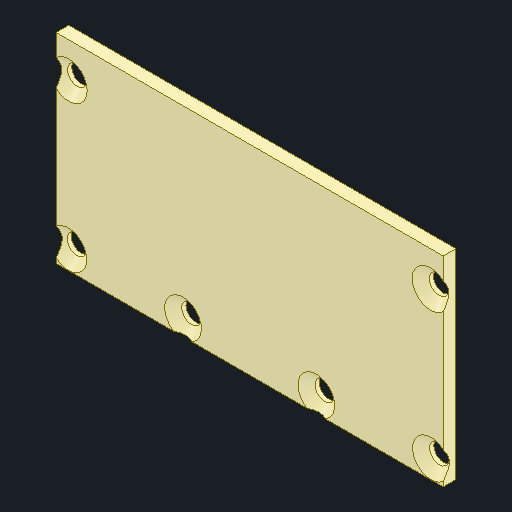
# Autodesk Inventor part: back
Saved by Autodesk Inventor 2023 (Build 270158000, 158)
## iProperties
Created: 2024-05-19
Part Number: back
Material: Nylon 6/6
Document SubType Name: Modeling
Designer: szymo
Density: 1.13 g/cm^3
Appearance: Nylon 6
Mass: 3.55753 g
Surface Area: 44.8899 cm^2
Volume: 3.14826 cm^3
Author: szymo
Autodesk Inventor part; units mm, degrees
ref_plane "YZ Plane" through (0, 0, 0) normal (1, 0, 0) x (0, 1, 0)
ref_plane "XZ Plane" through (0, 0, 0) normal (0, 1, 0) x (-1, 0, 0)
ref_plane "XY Plane" through (0, 0, 0) normal (0, 0, 1) x (1, 0, 0)
ref_plane "Work Plane1" through (22, 31.5, 0) normal (0, 0, 1) x (0, 1, 0)
sketch "Sketch1" plane through (22, 31.5, 0) normal (0, 0, 1) x (0, 1, 0)
  line L0 (0, 0) -> (0, 61) projected
  line L1 (0, 61) -> (-3.5, 61) projected
  line L2 (-3.5, 0) -> (-3.5, 61) projected
  circle A0 centre (-5.5, 2) radius 1.75 projected
  circle A1 centre (-28.5, 2) radius 1.75 projected
  line L3 (-3.5, 4) -> (-7.5, 4) projected
  arc A2 (-8.5, 3) -> (-7.5, 4) centre (-8.5, 4) ccw projected
  line L4 (-8.5, 3) -> (-21.7679, 3) projected
  arc A3 (-23.5, 4) -> (-21.7679, 3) centre (-21.7679, 5) ccw projected
  line L5 (-23.5, 4) -> (-31.5, 4) projected
  line L6 (-31.5, 0) -> (-31.5, 4) projected
  line L7 (-3.5, 0) -> (-3.5, 4) projected
  line L8 (-23.5, 22) -> (-3.5, 22) projected
  line L9 (-3.5, 22) -> (-3.5, 18) projected
  line L10 (-23.5, 39) -> (-3.5, 39) projected
  line L11 (-3.5, 39) -> (-3.5, 43) projected
  line L12 (-3.5, 57) -> (-6.7679, 57) projected
  line L13 (-3.5, 61) -> (-3.5, 57) projected
  line L14 (-3.5, 61) -> (-31.5, 61) projected
  line L15 (-31.5, 61) -> (-31.5, 57) projected
  line L16 (-24.004, 57) -> (-31.5, 57) projected
  line L17 (0, 0) -> (-31.5, 0)
  line L18 (-31.5, 0) -> (-31.5, 61)
  line L19 (-31.5, 61) -> (0, 61)
  line L20 (0, 61) -> (0, 0)
  line L21 (-3.5, 0) -> (-31.5, 0)
  line L22 (-8.5, 58) -> (-21.7679, 58) projected
  arc A4 (-7.634, 57.5) -> (-6.7679, 57) centre (-6.7679, 58) ccw projected
  arc A5 (-24.004, 57) -> (-23.2587, 57.3333) centre (-24.004, 58) ccw projected
  arc A6 (-21.7679, 58) -> (-23.2587, 57.3333) centre (-21.7679, 56) ccw projected
  arc A7 (-7.634, 57.5) -> (-8.5, 58) centre (-8.5, 57) ccw projected
  line L23 (-23.5, 18) -> (-23.5, 22) projected
  line L24 (-23.5, 18) -> (-3.5, 18) projected
  line L25 (-23.5, 43) -> (-3.5, 43) projected
  line L26 (-23.5, 43) -> (-23.5, 39) projected
  circle A8 centre (-5.5, 59) radius 1.75 projected
  circle A9 centre (-28.5, 59) radius 1.75 projected
  point P0 (-3.5, 28.5)
  point P1 (-3.5, 32.5)
  point P2 (-3.5, 61)
  point P3 (-13.5, 58)
  dimension "d25" = 0
  dimension "d26" = 0
  constraints: 10 end point, 1 horizontal, 1 parallel, 1 perpendicular, 1 vertical, 1 other
  measures "d25" distance between parallel lines of L19 L1
  measures "d26" distance from line of point (-3.5, 0) L17
extrude "Extrusion1" add sketch "Sketch1" along normal blind 2 contours L17 L2 L1 L0 | L17 L6 L5 A3 L4 A2 L3 L2 | L2 L12 A4 A7 L22 A6 A5 L16 L15 L14 | L3 A2 L4 A3 L5 L18 L16 A5 A6 L22 A7 A4 L12 L2 L25 L26 L10 L8 L23 L24 | L24 L23 L8 L2 | L2 L10 L26 L25 | A0 | A1 | A8 | A9
hole "Hole1" at (20.0645, 2.9032, 2) at (20, 26, 2) at (2, 2.5, 2) at (-19, 2.5, 2) at (-37, 26, 2) at (-37.0645, 2.9032, 2) direction (0, 0, -1) diameter 3.1 end through all countersink diameter 5.8 countersink angle 90 clearance for "Countersunk Flat Head Screw ISO 2009/7046" size "M2.5" standard "ISO"
sketch "Sketch4" plane through (22, 31.5, 0) normal (0, 0, -1) x (-1, 0, 0)
  line L0 (39, -23.5) -> (39, -3.5)
  line L1 (39, -3.5) -> (43, -3.5)
  line L2 (43, -23.5) -> (43, -3.5)
  line L3 (43, -23.5) -> (39, -23.5)
  line L4 (22, -23.5) -> (22, -3.5)
  line L5 (18, -23.5) -> (22, -23.5)
  line L6 (18, -23.5) -> (18, -3.5)
  line L7 (22, -3.5) -> (18, -3.5)
  circle A0 centre (20, -29) radius 1.75
  line L8 (22, -31.5) -> (18, -31.5)
  line L9 (18, -31.5) -> (18, -23.5)
  line L10 (22, -23.5) -> (18, -23.5)
  line L11 (22, -23.5) -> (22, -31.5)
  circle A1 centre (41, -29) radius 1.75
  line L12 (39, -31.5) -> (43, -31.5)
  line L13 (39, -23.5) -> (39, -31.5)
  line L14 (39, -23.5) -> (43, -23.5)
  line L15 (43, -31.5) -> (43, -23.5)
  circle A2 centre (59, -5.5) radius 1.75
  circle A3 centre (59, -28.5) radius 1.75
  arc A4 (57, -6.7679) -> (57.5, -7.634) centre (58, -6.7679) ccw
  line L16 (57, -3.5) -> (57, -6.7679)
  line L17 (61, -3.5) -> (57, -3.5)
  line L18 (61, -3.5) -> (61, -31.5)
  line L19 (61, -31.5) -> (57, -31.5)
  line L20 (57, -24.004) -> (57, -31.5)
  arc A5 (57.3333, -23.2587) -> (57, -24.004) centre (58, -24.004) ccw
  arc A6 (57.3333, -23.2587) -> (58, -21.7679) centre (56, -21.7679) ccw
  line L21 (58, -8.5) -> (58, -21.7679)
  arc A7 (58, -8.5) -> (57.5, -7.634) centre (57, -8.5) ccw
  line L22 (61, -31.5) -> (42.4697, -31.5)
  line L23 (0, -31.5) -> (0, 0)
  line L24 (61, -31.5) -> (0, -31.5)
  line L25 (0, -31.5) -> (0, -25.5)
  line L26 (0, -25.5) -> (61, -25.5)
  line L27 (61, -25.5) -> (61, -31.5)
  line L28 (61, 0) -> (61, -31.5)
  line L29 (0, -8.5) -> (61, -8.5)
  line L30 (61, -8.5) -> (61, -2.5)
  line L31 (61, -2.5) -> (0, -2.5)
  line L32 (0, -2.5) -> (0, -8.5)
  circle A8 centre (41, -29) radius 1.55
  line L33 (59, -5.5) -> (41, -29) construction
  line L34 (2, -5.5) -> (20, -29) construction
  arc A9 (42.4697, -31.5) -> (39.5303, -31.5) centre (41, -29) ccw
  line L35 (41, -29) -> (30.5, -8.5) construction
  line L36 (20, -29) -> (30.5, -8.5) construction
  circle A10 centre (1.9355, -28.5968) radius 1.55
  line L37 (57, -25.5) -> (57, -8.5)
  line L38 (4, -25.5) -> (4, -8.5)
  line L39 (57, -10.5779) -> (45.5703, -25.5)
  line L40 (54.8127, -8.5) -> (41.7914, -25.5)
  line L41 (40.8926, -25.5) -> (32.1853, -8.5)
  line L42 (28.8147, -8.5) -> (20.1817, -25.3548)
  line L43 (23.478, -25.5) -> (30.5, -11.7904)
  line L44 (30.5, -11.7904) -> (37.522, -25.5)
  line L45 (19.2086, -25.5) -> (6.1873, -8.5)
  line L46 (4, -10.5779) -> (15.4297, -25.5)
  arc A11 (21.4697, -31.5) -> (18.5303, -31.5) centre (20, -29) ccw
  line L47 (18.5303, -31.5) -> (0, -31.5)
  line L48 (0, -31.5) -> (0, -30.7564)
  line L49 (0, 0) -> (61, 0)
  line L50 (61, 0) -> (61, -3.4)
  line L51 (61, -31.5) -> (42.4697, -31.5)
  arc A12 (42.4697, -31.5) -> (39.5303, -31.5) centre (41, -29) ccw
  line L52 (39.5303, -31.5) -> (21.4697, -31.5)
  arc A13 (61, -26.4372) -> (61, -30.7564) centre (59.0645, -28.5968) ccw
  arc A14 (0, -7.6) -> (0, -3.4) centre (2, -5.5) ccw
  arc A15 (0, -30.7564) -> (0, -26.4372) centre (1.9355, -28.5968) ccw
  arc A16 (61, -3.4) -> (61, -7.6) centre (59, -5.5) ccw
  line L53 (61, -7.6) -> (61, -26.4372)
  line L54 (61, -30.7564) -> (61, -31.5)
  line L55 (0, -26.4372) -> (0, -7.6)
  line L56 (0, -3.4) -> (0, 0)
  line L57 (61, -3.5) -> (57, -3.5)
  line L58 (61, -3.5) -> (61, -31.5)
  line L59 (61, -31.5) -> (57, -31.5)
  line L60 (57, -3.5) -> (57, -31.5)
  point P0 (18, -23.9221)
  point P1 (18, -8.5)
  point P2 (22, -21.8049)
  point P3 (22, -8.5)
  point P4 (39, -21.8049)
  point P5 (39, -8.5)
  point P6 (43, -23.9221)
  point P7 (43, -8.5)
  point P8 (0, -2.5)
extrude "Extrusion3" cut sketch "Sketch4" against normal blind 1 contours L41 L29 L0 | L2 L29 L40 L15 | L26 L43 L44 | L42 L4 L29 | L6 L9 L45 L29 | L39 L37 L20 L26 | L26 L38 L46
body "Solid1"
